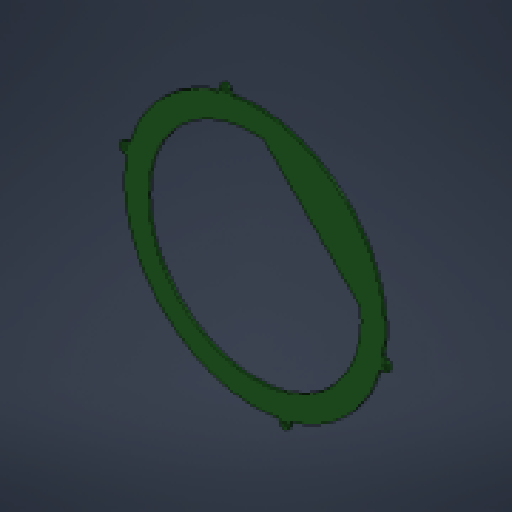
# Autodesk Inventor part: LineSensor
Saved by Autodesk Inventor 2024.2 (Build 282272000, 272)
## iProperties
Created: 2023-12-21
Part Number: LineSensor
Material: 一般
Document SubType Name: Modeling
Designer: Hanaoka
Density: 1 g/cm^3
Appearance: 既定
Author: Hanaoka
Autodesk Inventor part; units mm, degrees
ref_plane "YZ Plane" through (0, 0, 0) normal (1, 0, 0) x (0, 1, 0)
ref_plane "XZ Plane" through (0, 0, 0) normal (0, 1, 0) x (-1, 0, 0)
ref_plane "作業平面1" through (0, 0, 0) normal (0, 0, 1) x (1, 0, 0)
sketch "スケッチ1" plane through (0, 0, 0) normal (0, 0, 1) x (1, 0, 0)
  circle A0 centre (-14.624772, 63.539385) radius 64
  arc A1 (-81.893775, 52.547912) -> (-80.479561, 53.962126) centre (-81.186668, 53.255019) ccw
  line L0 (-81.893775, 52.547912) -> (-83.065348, 52.547912)
  arc A2 (-84.479561, 53.962126) -> (-83.065348, 52.547912) centre (-83.772455, 53.255019) ccw
  line L1 (-84.479561, 53.962126) -> (-84.479561, 73.133699)
  arc A3 (-83.065348, 74.547912) -> (-84.479561, 73.133699) centre (-83.772455, 73.840806) ccw
  line L2 (-83.065348, 74.547912) -> (-81.893775, 74.547912)
  arc A4 (-80.479561, 73.133699) -> (-81.893775, 74.547912) centre (-81.186668, 73.840806) ccw
  line L3 (-80.479561, 73.133699) -> (-80.479561, 53.962126)
  arc A5 (-3.479561, 132.133699) -> (-4.893775, 133.547912) centre (-4.186668, 132.840806) ccw
  line L4 (-3.479561, 132.133699) -> (-3.479561, 130.962126)
  arc A6 (-4.893775, 129.547912) -> (-3.479561, 130.962126) centre (-4.186668, 130.255019) ccw
  line L5 (-4.893775, 129.547912) -> (-24.065348, 129.547912)
  arc A7 (-25.479561, 130.962126) -> (-24.065348, 129.547912) centre (-24.772455, 130.255019) ccw
  line L6 (-25.479561, 130.962126) -> (-25.479561, 132.133699)
  arc A8 (-24.065348, 133.547912) -> (-25.479561, 132.133699) centre (-24.772455, 132.840806) ccw
  line L7 (-24.065348, 133.547912) -> (-4.893775, 133.547912)
  arc A9 (54.106225, 52.547912) -> (55.520439, 53.962126) centre (54.813332, 53.255019) ccw
  line L8 (54.106225, 52.547912) -> (52.934652, 52.547912)
  arc A10 (51.520439, 53.962126) -> (52.934652, 52.547912) centre (52.227545, 53.255019) ccw
  line L9 (51.520439, 53.962126) -> (51.520439, 73.133699)
  arc A11 (52.934652, 74.547912) -> (51.520439, 73.133699) centre (52.227545, 73.840806) ccw
  line L10 (52.934652, 74.547912) -> (54.106225, 74.547912)
  arc A12 (55.520439, 73.133699) -> (54.106225, 74.547912) centre (54.813332, 73.840806) ccw
  line L11 (55.520439, 73.133699) -> (55.520439, 53.962126)
  arc A13 (-25.479561, -5.037874) -> (-24.065348, -6.452088) centre (-24.772455, -5.744981) ccw
  line L12 (-25.479561, -5.037874) -> (-25.479561, -3.866301)
  arc A14 (-24.065348, -2.452088) -> (-25.479561, -3.866301) centre (-24.772455, -3.159194) ccw
  line L13 (-24.065348, -2.452088) -> (-4.893775, -2.452088)
  arc A15 (-3.479561, -3.866301) -> (-4.893775, -2.452088) centre (-4.186668, -3.159194) ccw
  line L14 (-3.479561, -3.866301) -> (-3.479561, -5.037874)
  arc A16 (-4.893775, -6.452088) -> (-3.479561, -5.037874) centre (-4.186668, -5.744981) ccw
  line L15 (-4.893775, -6.452088) -> (-24.065348, -6.452088)
  arc A17 (-90.380937, 104.093949) -> (-92.776199, 103.718007) centre (-91.441598, 103.033289) ccw
  arc A18 (-92.776199, 103.718007) -> (-98.248191, 90.50745) centre (-14.479561, 63.547912) ccw
  arc A19 (-98.248191, 90.50745) -> (-96.820317, 88.547912) centre (-96.820317, 90.047912) ccw
  line L16 (-96.820317, 88.547912) -> (-88.479561, 88.547912)
  arc A20 (-86.479561, 86.547912) -> (-88.479561, 88.547912) centre (-88.479561, 86.547912) ccw
  line L17 (-86.479561, 86.547912) -> (-86.479561, 40.547912)
  arc A21 (-88.479561, 38.547912) -> (-86.479561, 40.547912) centre (-88.479561, 40.547912) ccw
  line L18 (-88.479561, 38.547912) -> (-96.820317, 38.547912)
  arc A22 (-96.820317, 38.547912) -> (-98.248191, 36.588375) centre (-96.820317, 37.047912) ccw
  arc A23 (-98.248191, 36.588375) -> (-41.439099, -20.220717) centre (-14.479561, 63.547912) ccw
  arc A24 (-41.439099, -20.220717) -> (-39.479561, -18.792843) centre (-40.979561, -18.792843) ccw
  line L19 (-39.479561, -18.792843) -> (-39.479561, -10.452088)
  arc A25 (-37.479561, -8.452088) -> (-39.479561, -10.452088) centre (-37.479561, -10.452088) ccw
  line L20 (-37.479561, -8.452088) -> (8.520439, -8.452088)
  arc A26 (10.520439, -10.452088) -> (8.520439, -8.452088) centre (8.520439, -10.452088) ccw
  line L21 (10.520439, -10.452088) -> (10.520439, -18.792843)
  arc A27 (10.520439, -18.792843) -> (12.479976, -20.220717) centre (12.020439, -18.792843) ccw
  arc A28 (12.479976, -20.220717) -> (25.690533, -14.748726) centre (-14.479561, 63.547912) ccw
  arc A29 (25.690533, -14.748726) -> (26.066476, -12.353464) centre (25.005815, -13.414124) ccw
  line L22 (26.066476, -12.353464) -> (20.079693, -6.366681)
  arc A30 (20.079693, -2.124041) -> (20.079693, -6.366681) centre (22.201014, -4.245361) ccw
  line L23 (25.736548, 3.532814) -> (45.535537, 23.331803)
  arc A31 (55.435032, 28.988658) -> (51.192392, 28.988658) centre (53.313712, 26.867337) ccw
  line L24 (55.435032, 28.988658) -> (61.421815, 23.001875)
  arc A32 (61.421815, 23.001875) -> (63.817077, 23.377818) centre (62.482475, 24.062536) ccw
  arc A33 (63.817077, 23.377818) -> (69.289068, 36.588375) centre (-14.479561, 63.547912) ccw
  arc A34 (69.289068, 36.588375) -> (67.861194, 38.547912) centre (67.861194, 37.047912) ccw
  line L25 (67.861194, 38.547912) -> (59.520439, 38.547912)
  arc A35 (57.520439, 40.547912) -> (59.520439, 38.547912) centre (59.520439, 40.547912) ccw
  line L26 (57.520439, 40.547912) -> (57.520439, 86.547912)
  arc A36 (59.520439, 88.547912) -> (57.520439, 86.547912) centre (59.520439, 86.547912) ccw
  line L27 (59.520439, 88.547912) -> (67.861194, 88.547912)
  arc A37 (67.861194, 88.547912) -> (69.289068, 90.50745) centre (67.861194, 90.047912) ccw
  arc A38 (69.289068, 90.50745) -> (12.479976, 147.316542) centre (-14.479561, 63.547912) ccw
  arc A39 (12.479976, 147.316542) -> (10.520439, 145.888668) centre (12.020439, 145.888668) ccw
  line L28 (10.520439, 145.888668) -> (10.520439, 137.547912)
  arc A40 (8.520439, 135.547912) -> (10.520439, 137.547912) centre (8.520439, 137.547912) ccw
  line L29 (8.520439, 135.547912) -> (-37.479561, 135.547912)
  arc A41 (-39.479561, 137.547912) -> (-37.479561, 135.547912) centre (-37.479561, 137.547912) ccw
  line L30 (-39.479561, 137.547912) -> (-39.479561, 145.888668)
  arc A42 (-39.479561, 145.888668) -> (-41.439099, 147.316542) centre (-40.979561, 145.888668) ccw
  arc A43 (-41.439099, 147.316542) -> (-54.649656, 141.84455) centre (-14.479561, 63.547912) ccw
  arc A44 (-54.649656, 141.84455) -> (-55.025598, 139.449288) centre (-53.964938, 140.509949) ccw
  line L31 (-55.025598, 139.449288) -> (-49.038816, 133.462506)
  arc A45 (-49.038816, 129.219865) -> (-49.038816, 133.462506) centre (-51.160136, 131.341186) ccw
  line L32 (-49.038816, 129.219865) -> (-51.160136, 127.098545)
  arc A46 (-84.394155, 98.107167) -> (-80.151514, 98.107167) centre (-82.272835, 100.228487) ccw
  line L33 (-84.394155, 98.107167) -> (-90.380937, 104.093949)
  arc A47 (-32.657783, 124.912008) -> (-31.62228, 126.687656) centre (-33.083835, 126.350229) ccw
  line L34 (-31.62228, 126.687656) -> (-31.649781, 126.806774)
  arc A48 (-26.77793, 127.931529) -> (-31.649781, 126.806774) centre (-29.213855, 127.369152) ccw
  line L35 (-26.77793, 127.931529) -> (-26.75043, 127.812411)
  arc A49 (-26.75043, 127.812411) -> (-25.041333, 126.670404) centre (-25.288875, 128.149838) ccw
  arc A50 (48.642931, 52.986141) -> (-25.041333, 126.670404) centre (-14.479561, 63.547912) ccw
  arc A51 (48.642931, 52.986141) -> (49.784937, 51.277044) centre (50.122364, 52.738599) ccw
  line L36 (49.784937, 51.277044) -> (49.904056, 51.249544)
  arc A52 (48.7793, 46.377693) -> (49.904056, 51.249544) centre (49.341678, 48.813618) ccw
  line L37 (48.7793, 46.377693) -> (48.660182, 46.405194)
  arc A53 (48.660182, 46.405194) -> (46.884535, 45.369691) centre (48.322756, 44.943639) ccw
  arc A54 (3.69866, 2.183817) -> (46.884535, 45.369691) centre (-14.479561, 63.547912) ccw
  arc A55 (3.69866, 2.183817) -> (2.663157, 0.408169) centre (4.124712, 0.745596) ccw
  line L38 (2.663157, 0.408169) -> (2.690658, 0.289051)
  arc A56 (-2.181192, -0.835704) -> (2.690658, 0.289051) centre (0.254733, -0.273327) ccw
  line L39 (-2.181192, -0.835704) -> (-2.208693, -0.716586)
  arc A57 (-2.208693, -0.716586) -> (-3.91779, 0.425421) centre (-3.670248, -1.054013) ccw
  arc A58 (-77.602053, 74.109684) -> (-3.91779, 0.425421) centre (-14.479561, 63.547912) ccw
  arc A59 (-77.602053, 74.109684) -> (-78.74406, 75.818781) centre (-79.081487, 74.357226) ccw
  line L40 (-78.74406, 75.818781) -> (-78.863178, 75.846281)
  arc A60 (-77.738423, 80.718132) -> (-78.863178, 75.846281) centre (-78.300801, 78.282206) ccw
  line L41 (-77.738423, 80.718132) -> (-77.619305, 80.690631)
  arc A61 (-77.619305, 80.690631) -> (-75.843657, 81.726134) centre (-77.281878, 82.152186) ccw
  arc A62 (-32.657783, 124.912008) -> (-75.843657, 81.726134) centre (-14.479561, 63.547912) ccw
  circle A63 centre (65.069166, 92.047912) radius 2.5
  circle A64 centre (-42.979561, -16.000815) radius 2.5
  circle A65 centre (14.020439, 143.09664) radius 2.5
  circle A66 centre (-94.028289, 35.047912) radius 2.5
  circle A67 centre (49.341678, 48.813618) radius 1
  circle A68 centre (0.254733, -0.273327) radius 1
  circle A69 centre (-78.300801, 78.282206) radius 1
  circle A70 centre (-29.213855, 127.369152) radius 1
  circle A71 centre (-14.479561, 63.547912) radius 52.5
  circle A72 centre (19.135053, 141.074087) radius 2
  circle A73 centre (63.046613, 97.162527) radius 2
  circle A74 centre (2.020439, 127.968406) radius 2
  circle A75 centre (49.940932, 80.047912) radius 2
  line L42 (-74.49466, 103.056915) -> (-72.019786, 100.582041)
  line L43 (-71.31268, 99.874934) -> (-74.141107, 97.046507)
  line L44 (-74.848214, 97.753614) -> (-77.323087, 100.228487)
  line L45 (-54.69567, 123.563011) -> (-74.49466, 103.764021)
  line L46 (-51.160136, 126.391438) -> (-48.685263, 123.916565)
  line L47 (-47.978156, 123.209458) -> (-50.806583, 120.381031)
  line L48 (-51.51369, 121.088137) -> (-53.988563, 123.563011)
  arc A76 (-47.978156, 123.209458) -> (-48.685263, 123.916565) centre (-48.331709, 123.563011) ccw
  arc A77 (-51.51369, 121.088137) -> (-50.806583, 120.381031) centre (-51.160136, 120.734584) ccw
  arc A78 (-71.31268, 99.874934) -> (-72.019786, 100.582041) centre (-71.666233, 100.228487) ccw
  arc A79 (-74.848214, 97.753614) -> (-74.141107, 97.046507) centre (-74.49466, 97.40006) ccw
  line L49 (-78.030194, 100.228487) -> (-80.151514, 98.107167)
  line L50 (22.201014, 0.704386) -> (19.72614, 3.17926)
  arc A80 (19.019033, 3.886367) -> (19.72614, 3.17926) centre (19.372587, 3.532814) ccw
  line L51 (19.019033, 3.886367) -> (21.84746, 6.714794)
  arc A81 (22.554567, 6.007687) -> (21.84746, 6.714794) centre (22.201014, 6.361241) ccw
  line L52 (22.554567, 6.007687) -> (25.029441, 3.532814)
  line L53 (49.071071, 26.867337) -> (51.192392, 28.988658)
  line L54 (45.535537, 24.03891) -> (43.060664, 26.513784)
  arc A82 (42.353557, 27.220891) -> (43.060664, 26.513784) centre (42.70711, 26.867337) ccw
  line L55 (42.353557, 27.220891) -> (45.181984, 30.049318)
  arc A83 (45.889091, 29.342211) -> (45.181984, 30.049318) centre (45.535537, 29.695765) ccw
  line L56 (45.889091, 29.342211) -> (48.363965, 26.867337)
  line L57 (20.079693, -2.124041) -> (22.201014, -0.00272)
  arc A84 (22.201014, -0.00272) -> (22.201014, 0.704386) centre (21.84746, 0.350833) ccw
  arc A85 (25.029441, 3.532814) -> (25.736548, 3.532814) centre (25.382994, 3.886367) ccw
  arc A86 (45.535537, 23.331803) -> (45.535537, 24.03891) centre (45.181984, 23.685357) ccw
  arc A87 (48.363965, 26.867337) -> (49.071071, 26.867337) centre (48.717518, 27.220891) ccw
  arc A88 (-51.160136, 127.098545) -> (-51.160136, 126.391438) centre (-50.806583, 126.744992) ccw
  arc A89 (-53.988563, 123.563011) -> (-54.69567, 123.563011) centre (-54.342117, 123.209458) ccw
  arc A90 (-74.49466, 103.764021) -> (-74.49466, 103.056915) centre (-74.141107, 103.410468) ccw
  arc A91 (-77.323087, 100.228487) -> (-78.030194, 100.228487) centre (-77.676641, 99.874934) ccw
  arc A92 (30.422034, 111.235402) -> (31.814662, 111.256349) centre (31.107555, 111.963456) ccw
  arc A93 (30.422034, 111.235402) -> (5.557839, 125.907776) centre (-14.479561, 63.547912) ccw
  arc A94 (4.902925, 127.136978) -> (5.557839, 125.907776) centre (5.863754, 126.859835) ccw
  arc A95 (4.902925, 127.136978) -> (2.020439, 130.968406) centre (2.020439, 127.968406) ccw
  line L58 (2.020439, 130.968406) -> (-0.686668, 130.968406)
  arc A96 (-1.686668, 131.968406) -> (-0.686668, 130.968406) centre (-0.686668, 131.968406) ccw
  line L59 (-1.686668, 131.968406) -> (-1.686668, 133.047912)
  arc A97 (-0.686668, 134.047912) -> (-1.686668, 133.047912) centre (-0.686668, 133.047912) ccw
  line L60 (-0.686668, 134.047912) -> (11.020439, 134.047912)
  arc A98 (11.020439, 134.047912) -> (12.020439, 135.047912) centre (11.020439, 135.047912) ccw
  line L61 (12.020439, 135.047912) -> (12.020439, 138.179207)
  arc A99 (13.302114, 139.138717) -> (12.020439, 138.179207) centre (13.020439, 138.179207) ccw
  line L62 (13.302114, 139.138717) -> (18.14919, 137.715802)
  arc A100 (18.14919, 137.715802) -> (22.557489, 140.341331) centre (19.135053, 141.074087) ccw
  arc A101 (23.979947, 141.027692) -> (22.557489, 140.341331) centre (23.535328, 140.131972) ccw
  arc A102 (45.237685, 126.126667) -> (23.979947, 141.027692) centre (-14.479561, 63.547912) ccw
  arc A103 (45.254419, 124.696106) -> (45.237685, 126.126667) centre (44.547312, 125.403213) ccw
  line L63 (45.254419, 124.696106) -> (31.814662, 111.256349)
  arc A104 (55.020439, 76.340806) -> (56.020439, 77.340806) centre (55.020439, 77.340806) ccw
  line L64 (55.020439, 76.340806) -> (53.940932, 76.340806)
  arc A105 (52.940932, 77.340806) -> (53.940932, 76.340806) centre (53.940932, 77.340806) ccw
  line L65 (52.940932, 77.340806) -> (52.940932, 80.047912)
  arc A106 (52.940932, 80.047912) -> (49.109504, 82.930399) centre (49.940932, 80.047912) ccw
  arc A107 (47.880302, 83.585313) -> (49.109504, 82.930399) centre (48.832361, 83.891227) ccw
  arc A108 (47.880302, 83.585313) -> (33.207929, 108.449508) centre (-14.479561, 63.547912) ccw
  arc A109 (33.228875, 109.842135) -> (33.207929, 108.449508) centre (33.935982, 109.135029) ccw
  line L66 (33.228875, 109.842135) -> (46.668632, 123.281893)
  arc A110 (48.099193, 123.265159) -> (46.668632, 123.281893) centre (47.375739, 122.574786) ccw
  arc A111 (63.000218, 102.00742) -> (48.099193, 123.265159) centre (-14.479561, 63.547912) ccw
  arc A112 (62.313857, 100.584963) -> (63.000218, 102.00742) centre (62.104498, 101.562802) ccw
  arc A113 (62.313857, 100.584963) -> (59.688329, 96.176664) centre (63.046613, 97.162527) ccw
  line L67 (59.688329, 96.176664) -> (61.111243, 91.329587)
  arc A114 (60.151733, 90.047912) -> (61.111243, 91.329587) centre (60.151733, 91.047912) ccw
  line L68 (60.151733, 90.047912) -> (57.020439, 90.047912)
  arc A115 (57.020439, 90.047912) -> (56.020439, 89.047912) centre (57.020439, 89.047912) ccw
  line L69 (56.020439, 89.047912) -> (56.020439, 77.340806)
  arc A116 (54.874372, 32.670638) -> (54.874372, 31.670638) centre (54.874372, 32.170638) ccw
  line L70 (54.874372, 32.670638) -> (56.702799, 34.499065)
  arc A117 (57.702799, 34.499065) -> (56.702799, 34.499065) centre (57.202799, 34.499065) ccw
  line L71 (57.702799, 34.499065) -> (62.359654, 29.842211)
  arc A118 (62.359654, 28.842211) -> (62.359654, 29.842211) centre (62.359654, 29.342211) ccw
  line L72 (62.359654, 28.842211) -> (60.531226, 27.013784)
  arc A119 (59.531226, 27.013784) -> (60.531226, 27.013784) centre (60.031226, 27.013784) ccw
  line L73 (59.531226, 27.013784) -> (54.874372, 31.670638)
  arc A120 (-86.661922, 92.596759) -> (-85.661922, 92.596759) centre (-86.161922, 92.596759) ccw
  line L74 (-86.661922, 92.596759) -> (-91.318776, 97.253614)
  arc A121 (-91.318776, 98.253614) -> (-91.318776, 97.253614) centre (-91.318776, 97.753614) ccw
  line L75 (-91.318776, 98.253614) -> (-89.490349, 100.082041)
  arc A122 (-88.490349, 100.082041) -> (-89.490349, 100.082041) centre (-88.990349, 100.082041) ccw
  line L76 (-88.490349, 100.082041) -> (-83.833495, 95.425187)
  arc A123 (-83.833495, 94.425187) -> (-83.833495, 95.425187) centre (-83.833495, 94.925187) ccw
  line L77 (-83.833495, 94.425187) -> (-85.661922, 92.596759)
  line L78 (19.22614, -13.291303) -> (14.569286, -8.634448)
  arc A124 (14.569286, -7.634448) -> (14.569286, -8.634448) centre (14.569286, -8.134448) ccw
  line L79 (14.569286, -7.634448) -> (16.397713, -5.806021)
  arc A125 (17.397713, -5.806021) -> (16.397713, -5.806021) centre (16.897713, -5.806021) ccw
  line L80 (17.397713, -5.806021) -> (22.054567, -10.462875)
  arc A126 (22.054567, -11.462875) -> (22.054567, -10.462875) centre (22.054567, -10.962875) ccw
  line L81 (22.054567, -11.462875) -> (20.22614, -13.291303)
  arc A127 (19.22614, -13.291303) -> (20.22614, -13.291303) centre (19.72614, -13.291303) ccw
  line L82 (-48.185263, 140.387127) -> (-43.528408, 135.730273)
  arc A128 (-43.528408, 134.730273) -> (-43.528408, 135.730273) centre (-43.528408, 135.230273) ccw
  line L83 (-43.528408, 134.730273) -> (-45.356835, 132.901846)
  arc A129 (-46.356835, 132.901846) -> (-45.356835, 132.901846) centre (-45.856835, 132.901846) ccw
  line L84 (-46.356835, 132.901846) -> (-51.01369, 137.5587)
  arc A130 (-51.01369, 138.5587) -> (-51.01369, 137.5587) centre (-51.01369, 138.0587) ccw
  line L85 (-51.01369, 138.5587) -> (-49.185263, 140.387127)
  arc A131 (-48.185263, 140.387127) -> (-49.185263, 140.387127) centre (-48.685263, 140.387127) ccw
  arc A132 (-1.686668, -5.952088) -> (-0.686668, -6.952088) centre (-0.686668, -5.952088) ccw
  line L86 (-1.686668, -5.952088) -> (-1.686668, -5.183904)
  arc A133 (-0.498388, -4.201788) -> (-1.686668, -5.183904) centre (-0.686668, -5.183904) ccw
  arc A134 (-0.498388, -4.201788) -> (4.246848, -0.022298) centre (0.254733, -0.273327) ccw
  arc A135 (4.948269, 0.995459) -> (4.246848, -0.022298) centre (5.244877, 0.04046) ccw
  arc A136 (4.948269, 0.995459) -> (14.374317, 4.74567) centre (-14.479561, 63.547912) ccw
  arc A137 (15.521941, 4.555032) -> (14.374317, 4.74567) centre (14.814834, 3.847926) ccw
  line L87 (15.521941, 4.555032) -> (19.372587, 0.704386)
  arc A138 (19.372587, -0.709827) -> (19.372587, 0.704386) centre (18.66548, -0.00272) ccw
  line L88 (19.372587, -0.709827) -> (13.423219, -6.659194)
  arc A139 (12.716112, -6.952088) -> (13.423219, -6.659194) centre (12.716112, -5.952088) ccw
  line L89 (12.716112, -6.952088) -> (-0.686668, -6.952088)
  arc A140 (-96.383203, 91.36955) -> (-95.43634, 90.047912) centre (-95.43634, 91.047912) ccw
  arc A141 (-94.512296, 96.365763) -> (-96.383203, 91.36955) centre (-14.479561, 63.547912) ccw
  arc A142 (-92.879956, 96.693473) -> (-94.512296, 96.365763) centre (-93.587062, 95.986366) ccw
  line L90 (-92.879956, 96.693473) -> (-87.941502, 91.755019)
  arc A143 (-88.648609, 90.047912) -> (-87.941502, 91.755019) centre (-88.648609, 91.047912) ccw
  line L91 (-88.648609, 90.047912) -> (-95.43634, 90.047912)
  arc A144 (-47.297412, 143.580647) -> (-47.625122, 141.948307) centre (-46.918015, 142.655414) ccw
  arc A145 (-42.301199, 145.451554) -> (-47.297412, 143.580647) centre (-14.479561, 63.547912) ccw
  arc A146 (-40.979561, 144.504691) -> (-42.301199, 145.451554) centre (-41.979561, 144.504691) ccw
  line L92 (-40.979561, 144.504691) -> (-40.979561, 137.71696)
  arc A147 (-42.686668, 137.009853) -> (-40.979561, 137.71696) centre (-41.979561, 137.71696) ccw
  line L93 (-42.686668, 137.009853) -> (-47.625122, 141.948307)
  arc A148 (67.42408, 35.726275) -> (66.477217, 37.047912) centre (66.477217, 36.047912) ccw
  arc A149 (65.553174, 30.730062) -> (67.42408, 35.726275) centre (-14.479561, 63.547912) ccw
  arc A150 (63.920833, 30.402352) -> (65.553174, 30.730062) centre (64.62794, 31.109459) ccw
  line L94 (63.920833, 30.402352) -> (58.982379, 35.340806)
  arc A151 (59.689486, 37.047912) -> (58.982379, 35.340806) centre (59.689486, 36.047912) ccw
  line L95 (59.689486, 37.047912) -> (66.477217, 37.047912)
  arc A152 (18.338289, -16.484823) -> (18.665999, -14.852482) centre (17.958892, -15.559589) ccw
  arc A153 (13.342076, -18.355729) -> (18.338289, -16.484823) centre (-14.479561, 63.547912) ccw
  arc A154 (12.020439, -17.408866) -> (13.342076, -18.355729) centre (13.020439, -17.408866) ccw
  line L96 (12.020439, -17.408866) -> (12.020439, -10.621135)
  arc A155 (13.727545, -9.914028) -> (12.020439, -10.621135) centre (13.020439, -10.621135) ccw
  line L97 (13.727545, -9.914028) -> (18.665999, -14.852482)
  arc A156 (-77.323087, 97.40006) -> (-78.737301, 97.40006) centre (-78.030194, 96.692954) ccw
  line L98 (-77.323087, 97.40006) -> (-73.472441, 93.549414)
  arc A157 (-73.281804, 92.40179) -> (-73.472441, 93.549414) centre (-74.179548, 92.842308) ccw
  arc A158 (-73.281804, 92.40179) -> (-77.032015, 82.975742) centre (-14.479561, 63.547912) ccw
  arc A159 (-78.049771, 82.274322) -> (-77.032015, 82.975742) centre (-77.987014, 83.272351) ccw
  arc A160 (-78.049771, 82.274322) -> (-82.229262, 77.529086) centre (-78.300801, 78.282206) ccw
  arc A161 (-83.211377, 76.340806) -> (-82.229262, 77.529086) centre (-83.211377, 77.340806) ccw
  line L99 (-83.211377, 76.340806) -> (-83.979561, 76.340806)
  arc A162 (-84.979561, 77.340806) -> (-83.979561, 76.340806) centre (-83.979561, 77.340806) ccw
  line L100 (-84.979561, 77.340806) -> (-84.979561, 90.743586)
  arc A163 (-84.686668, 91.450693) -> (-84.979561, 90.743586) centre (-83.979561, 90.743586) ccw
  line L101 (-84.686668, 91.450693) -> (-78.737301, 97.40006)
  arc A164 (-27.272455, 133.047912) -> (-28.272455, 134.047912) centre (-28.272455, 133.047912) ccw
  line L102 (-27.272455, 133.047912) -> (-27.272455, 132.279728)
  arc A165 (-28.460735, 131.297613) -> (-27.272455, 132.279728) centre (-28.272455, 132.279728) ccw
  arc A166 (-28.460735, 131.297613) -> (-33.205971, 127.118122) centre (-29.213855, 127.369152) ccw
  arc A167 (-33.907391, 126.100366) -> (-33.205971, 127.118122) centre (-34.203999, 127.055365) ccw
  arc A168 (-33.907391, 126.100366) -> (-43.333439, 122.350155) centre (-14.479561, 63.547912) ccw
  arc A169 (-44.481063, 122.540792) -> (-43.333439, 122.350155) centre (-43.773956, 123.247899) ccw
  line L103 (-44.481063, 122.540792) -> (-48.331709, 126.391438)
  arc A170 (-48.331709, 127.805652) -> (-48.331709, 126.391438) centre (-47.624602, 127.098545) ccw
  line L104 (-48.331709, 127.805652) -> (-42.382342, 133.755019)
  arc A171 (-41.675235, 134.047912) -> (-42.382342, 133.755019) centre (-41.675235, 133.047912) ccw
  line L105 (-41.675235, 134.047912) -> (-28.272455, 134.047912)
  line L106 (55.727545, 35.645132) -> (49.778178, 29.695765)
  arc A172 (48.363965, 29.695765) -> (49.778178, 29.695765) centre (49.071071, 30.402871) ccw
  line L107 (48.363965, 29.695765) -> (44.513319, 33.54641)
  arc A173 (44.322681, 34.694034) -> (44.513319, 33.54641) centre (45.220425, 34.253517) ccw
  arc A174 (44.322681, 34.694034) -> (48.072892, 44.120082) centre (-14.479561, 63.547912) ccw
  arc A175 (49.090649, 44.821503) -> (48.072892, 44.120082) centre (49.027891, 43.823474) ccw
  arc A176 (49.090649, 44.821503) -> (53.270139, 49.566739) centre (49.341678, 48.813618) ccw
  arc A177 (54.252255, 50.755019) -> (53.270139, 49.566739) centre (54.252255, 49.755019) ccw
  line L108 (54.252255, 50.755019) -> (55.020439, 50.755019)
  arc A178 (56.020439, 49.755019) -> (55.020439, 50.755019) centre (55.020439, 49.755019) ccw
  line L109 (56.020439, 49.755019) -> (56.020439, 36.352239)
  arc A179 (55.727545, 35.645132) -> (56.020439, 36.352239) centre (55.020439, 36.352239) ccw
  arc A180 (-77.058316, 3.830666) -> (-75.627755, 3.813932) centre (-76.334862, 4.521039) ccw
  arc A181 (-91.959341, 25.088404) -> (-77.058316, 3.830666) centre (-14.479561, 63.547912) ccw
  arc A182 (-91.27298, 26.510862) -> (-91.959341, 25.088404) centre (-91.063621, 25.533023) ccw
  arc A183 (-91.27298, 26.510862) -> (-88.647451, 30.919161) centre (-92.005736, 29.933298) ccw
  line L110 (-88.647451, 30.919161) -> (-90.070366, 35.766237)
  arc A184 (-89.110856, 37.047912) -> (-90.070366, 35.766237) centre (-89.110856, 36.047912) ccw
  line L111 (-89.110856, 37.047912) -> (-85.979561, 37.047912)
  arc A185 (-85.979561, 37.047912) -> (-84.979561, 38.047912) centre (-85.979561, 38.047912) ccw
  line L112 (-84.979561, 38.047912) -> (-84.979561, 49.755019)
  arc A186 (-83.979561, 50.755019) -> (-84.979561, 49.755019) centre (-83.979561, 49.755019) ccw
  line L113 (-83.979561, 50.755019) -> (-82.900055, 50.755019)
  arc A187 (-81.900055, 49.755019) -> (-82.900055, 50.755019) centre (-82.900055, 49.755019) ccw
  line L114 (-81.900055, 49.755019) -> (-81.900055, 47.047912)
  arc A188 (-81.900055, 47.047912) -> (-78.068627, 44.165426) centre (-78.900055, 47.047912) ccw
  arc A189 (-76.839425, 43.510512) -> (-78.068627, 44.165426) centre (-77.791484, 43.204597) ccw
  arc A190 (-76.839425, 43.510512) -> (-62.167051, 18.646317) centre (-14.479561, 63.547912) ccw
  arc A191 (-62.187998, 17.253689) -> (-62.167051, 18.646317) centre (-62.895105, 17.960796) ccw
  line L115 (-62.187998, 17.253689) -> (-75.627755, 3.813932)
  arc A192 (-33.862048, -0.041153) -> (-30.979561, -3.872581) centre (-30.979561, -0.872581) ccw
  line L116 (-30.979561, -3.872581) -> (-28.272455, -3.872581)
  arc A193 (-27.272455, -4.872581) -> (-28.272455, -3.872581) centre (-28.272455, -4.872581) ccw
  line L117 (-27.272455, -4.872581) -> (-27.272455, -5.952088)
  arc A194 (-28.272455, -6.952088) -> (-27.272455, -5.952088) centre (-28.272455, -5.952088) ccw
  line L118 (-28.272455, -6.952088) -> (-39.979561, -6.952088)
  arc A195 (-39.979561, -6.952088) -> (-40.979561, -7.952088) centre (-39.979561, -7.952088) ccw
  line L119 (-40.979561, -7.952088) -> (-40.979561, -11.083382)
  arc A196 (-42.261236, -12.042892) -> (-40.979561, -11.083382) centre (-41.979561, -11.083382) ccw
  line L120 (-42.261236, -12.042892) -> (-47.108313, -10.619977)
  arc A197 (-47.108313, -10.619977) -> (-51.516612, -13.245506) centre (-48.094176, -13.978262) ccw
  arc A198 (-52.939069, -13.931867) -> (-51.516612, -13.245506) centre (-52.494451, -13.036147) ccw
  arc A199 (-74.196808, 0.969158) -> (-52.939069, -13.931867) centre (-14.479561, 63.547912) ccw
  arc A200 (-74.213542, 2.399719) -> (-74.196808, 0.969158) centre (-73.506435, 1.692612) ccw
  line L121 (-74.213542, 2.399719) -> (-60.773784, 15.839476)
  arc A201 (-59.381157, 15.860422) -> (-60.773784, 15.839476) centre (-60.066678, 15.132369) ccw
  arc A202 (-59.381157, 15.860422) -> (-34.516962, 1.188049) centre (-14.479561, 63.547912) ccw
  arc A203 (-33.862048, -0.041153) -> (-34.516962, 1.188049) centre (-34.822876, 0.23599) ccw
  line L122 (-10.23952, 115.876414) -> (37.84894, 67.787954)
  line L123 (-64.595165, 113.663516) -> (35.636043, 13.432309) construction
  point P0 (0, 0)
  point P1 (30.775273, 108.802746)
  dimension "d0" = 2
  dimension "d3" = 105
  dimension "d4" = 24
  constraints: 6 centre point, 5 coincident, 4 end point, 4 equal radius, 3 point on circle, 2 midpoint, 1 parallel
  measures "d0" diameter of A70
  measures "d3" diameter of A71
  measures "d4" distance from line of point (30.775, 108.803) L122
sketch "スケッチ1 outline for 押し出し1" plane through (0, 0, 0) normal (0, 0, 1) x (1, 0, 0)
  line L0 (-78.863178, 75.846281) -> (-78.74406, 75.818781)
  arc A0 (-78.74406, 75.818781) -> (-77.602053, 74.109684) centre (-79.081487, 74.357226) cw
  arc A1 (-77.602053, 74.109684) -> (-3.91779, 0.425421) centre (-14.479561, 63.547912) ccw
  arc A2 (-3.91779, 0.425421) -> (-2.208693, -0.716586) centre (-3.670248, -1.054013) cw
  line L1 (-2.208693, -0.716586) -> (-2.181192, -0.835704)
  arc A3 (-2.181192, -0.835704) -> (2.690658, 0.289051) centre (0.254733, -0.273327) ccw
  line L2 (2.690658, 0.289051) -> (2.663157, 0.408169)
  arc A4 (2.663157, 0.408169) -> (3.69866, 2.183817) centre (4.124712, 0.745596) cw
  arc A5 (3.69866, 2.183817) -> (46.884535, 45.369691) centre (-14.479561, 63.547912) ccw
  arc A6 (46.884535, 45.369691) -> (48.660182, 46.405194) centre (48.322756, 44.943639) cw
  line L3 (48.660182, 46.405194) -> (48.7793, 46.377693)
  arc A7 (48.7793, 46.377693) -> (49.904056, 51.249544) centre (49.341678, 48.813618) ccw
  line L4 (49.904056, 51.249544) -> (49.784937, 51.277044)
  arc A8 (49.784937, 51.277044) -> (48.642931, 52.986141) centre (50.122364, 52.738599) cw
  arc A9 (48.642931, 52.986141) -> (-25.041333, 126.670404) centre (-14.479561, 63.547912) ccw
  arc A10 (-25.041333, 126.670404) -> (-26.75043, 127.812411) centre (-25.288875, 128.149838) cw
  line L5 (-26.75043, 127.812411) -> (-26.77793, 127.931529)
  arc A11 (-26.77793, 127.931529) -> (-31.649781, 126.806774) centre (-29.213855, 127.369152) ccw
  line L6 (-31.649781, 126.806774) -> (-31.62228, 126.687656)
  arc A12 (-31.62228, 126.687656) -> (-32.657783, 124.912008) centre (-33.083835, 126.350229) cw
  arc A13 (-32.657783, 124.912008) -> (-75.843657, 81.726134) centre (-14.479561, 63.547912) ccw
  arc A14 (-75.843657, 81.726134) -> (-77.619305, 80.690631) centre (-77.281878, 82.152186) cw
  line L7 (-77.619305, 80.690631) -> (-77.738423, 80.718132)
  arc A15 (-77.738423, 80.718132) -> (-78.863178, 75.846281) centre (-78.300801, 78.282206) ccw
  circle A16 centre (0.254733, -0.273327) radius 1
  arc A17 (37.84894, 67.787954) -> (-10.23952, 115.876414) centre (-14.479561, 63.547912) cw
  line L8 (-10.23952, 115.876414) -> (37.84894, 67.787954)
  circle A18 centre (49.341678, 48.813618) radius 1
  circle A19 centre (-78.300801, 78.282206) radius 1
  circle A20 centre (-29.213855, 127.369152) radius 1
extrude "押し出し1" add sketch "スケッチ1 outline for 押し出し1" along normal blind 1.2
